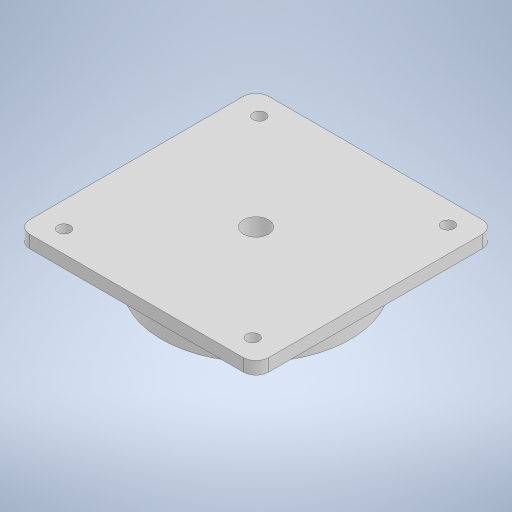
# Autodesk Inventor part: Saugknopf
Saved by Autodesk Inventor 2024 (Build 280153000, 153)
## iProperties
Created: 2023-11-16
Part Number: Saugknopf
Material: Generic
Document SubType Name: Modeling
Designer: Daniel Nussbaum
Density: 1 g/cm^3
Appearance: Default
Author: Daniel Nussbaum
Autodesk Inventor part; units mm, degrees
ref_plane "YZ Plane" through (0, 0, 0) normal (1, 0, 0) x (0, 1, 0)
ref_plane "XZ Plane" through (0, 0, 0) normal (0, 1, 0) x (-1, 0, 0)
ref_plane "XY Plane" through (0, 0, 0) normal (0, 0, 1) x (1, 0, 0)
sketch "Sketch1" plane through (0, 0, 0) normal (0, 1, 0) x (-1, 0, 0)
  circle A0 centre (0, 0) radius 37.5
  circle A1 centre (0, 0) radius 5
  dimension "d0" = 75
  dimension "d1" = 10
  constraints: 2 centre point, 2 coincident
  measures "d0" diameter of A0
  measures "d1" diameter of A1
extrude "Extrusion1" add sketch "Sketch1" along normal blind 15
sketch "Sketch2" plane through (0, 15, 0) normal (0, 1, 0) x (1, 0, 0)
  line L0 (-47.5, -47.5) -> (47.5, -47.5)
  line L1 (47.5, -47.5) -> (47.5, 47.5)
  line L2 (47.5, 47.5) -> (-47.5, 47.5)
  line L3 (-47.5, 47.5) -> (-47.5, -47.5)
  line L4 (-47.5, -47.5) -> (47.5, 47.5) construction
  line L5 (47.5, -47.5) -> (-47.5, 47.5) construction
  circle A0 centre (0, 0) radius 37.5 projected
  circle A1 centre (0, 0) radius 5 projected
  line L6 (-10, -5) -> (0, -5)
  line L7 (0, -5) -> (0, 5)
  line L8 (0, 5) -> (-10, 5)
  line L9 (-10, 5) -> (-10, -5)
  line L10 (-10, -5) -> (0, 5) construction
  line L11 (0, -5) -> (-10, 5) construction
  point P0 (-5, 0)
  dimension "d4" = 95
  dimension "d5" = 95
  constraints: 24 end point, 4 midpoint, 4 parallel, 2 horizontal, 2 perpendicular, 1 horizontal alignment, 1 other
  measures "d4" distance of L2.end L1.end
  measures "d5" distance of L1.end L0.end
extrude "Extrusion2" add sketch "Sketch2" along normal blind 5 contours L3 L2 L1 L0 | A0 | A1 L6 L9 L8
fillet "Fillet1" radius 5 4 edges at (47.5, 17.5, -47.5) (-47.5, 17.5, -47.5) (47.5, 17.5, 47.5) (-47.5, 17.5, 47.5)
sketch "Sketch4" plane through (0, 0, 0) normal (0, -1, 0) x (1, 0, 0)
  circle A0 centre (0, 0) radius 37.5 projected
  circle A1 centre (0, 0) radius 5 projected
  line L0 (0, 5) -> (-5, 5)
  line L1 (-5, 5) -> (-5, 0)
  line L2 (-5, -5) -> (0, -5)
  line L3 (-5, -5) -> (-5, 0)
  constraints: 8 end point, 3 point on circle, 2 perpendicular, 1 horizontal, 1 point on line
sketch "Sketch4 outline for Extrusion3" plane through (0, 0, 0) normal (0, -1, 0) x (1, 0, 0)
  line L0 (-5, 0) -> (-5, -5)
  arc A0 (0, -5) -> (-5, 0) centre (0, 0) cw
  line L1 (-5, -5) -> (0, -5)
  line L2 (-5, 5) -> (-5, 0)
  line L3 (0, 5) -> (-5, 5)
  arc A1 (-5, 0) -> (0, 5) centre (0, 0) cw
extrude "Extrusion3" cut sketch "Sketch4 outline for Extrusion3" against normal blind 10
sketch "Sketch6" plane through (0, 15, 0) normal (0, -1, 0) x (1, 0, 0)
  line L0 (37.5, 38.824232) -> (-37.5, 38.824232)
  line L1 (-37.5, 38.824232) -> (-37.5, -38.824232)
  line L2 (-37.5, -38.824232) -> (37.5, -38.824232)
  line L3 (37.5, -38.824232) -> (37.5, 38.824232)
  line L4 (37.5, 38.824232) -> (-37.5, -38.824232) construction
  line L5 (-37.5, 38.824232) -> (37.5, -38.824232) construction
  point P0 (0, 0)
  dimension "d11" = 75
  constraints: 12 end point, 4 coincident, 2 midpoint, 2 parallel, 1 horizontal, 1 perpendicular
  measures "d11" distance of L2.end L1.end
hole "Hole1" at (37.5, 15, -38.824232) at (-37.5, 15, -38.824232) at (-37.5, 15, 38.824232) at (37.5, 15, 38.824232) direction (0, 1, 0) diameter 5 end through all
body "Solid1"
